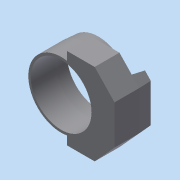
# Autodesk Inventor part: cellSTORM_inverted_objectiveadapter
Saved by Autodesk Inventor 2019.4 (Build 234330000, 330)
## iProperties
Created: 2020-11-10
Part Number: cellSTORM_inverted_objectiveadapter
Material: Generic
Document SubType Name: Modeling
Designer: diederichbenedict
Density: 1 g/cm^3
Appearance: Default
Author: diederichbenedict
Autodesk Inventor part; units mm, degrees
ref_plane "YZ Plane" through (0, 0, 0) normal (1, 0, 0) x (0, 1, 0)
ref_plane "XZ Plane" through (0, 0, 0) normal (0, 1, 0) x (-1, 0, 0)
ref_plane "XY Plane" through (0, 0, 0) normal (0, 0, 1) x (1, 0, 0)
sketch "Sketch1" plane through (0, 0, 0) normal (0, 0, 1) x (1, 0, 0)
  arc A0 (-5.5118, -5.25) -> (-5.5118, 21.75) centre (-8.0118, 8.25) ccw projected
  circle A1 centre (-7.8118, 8.25) radius 10 construction
  circle A2 centre (-7.8118, 8.25) radius 12.15 construction
  line L0 (-5.5118, -8.25) -> (-5.5118, -5.25) construction
  line L1 (7.4882, -8.25) -> (-5.5118, -8.25) construction
  line L2 (11.0118, -4.7265) -> (7.4882, -8.25) construction
  line L3 (11.0118, -4.7265) -> (11.0118, 21.2265) construction
  line L4 (11.0118, 21.2265) -> (7.4882, 24.75) construction
  line L5 (7.4882, 24.75) -> (-5.5118, 24.75) construction
  line L6 (-5.5118, 24.75) -> (-5.5118, 21.75) construction
  arc A3 (-5.5118, -5.25) -> (-5.5118, 21.75) centre (-8.0118, 8.25) ccw construction
  circle A4 centre (-7.8118, 8.25) radius 12.25
  circle A5 centre (-7.8118, 8.25) radius 13.25
  line L7 (-5.5118, 21.2989) -> (-5.5118, 24.75)
  line L8 (-5.5118, 24.75) -> (5.7178, 24.75)
  line L9 (5.7178, 24.75) -> (5.7178, -8.25)
  line L10 (5.7178, 24.75) -> (38.7178, 24.75) construction
  line L11 (5.7178, -8.25) -> (-5.5118, -8.25)
  line L12 (-5.5118, -8.25) -> (-5.5118, -4.7989)
  line L13 (13.7178, 16.3622) -> (5.7178, 16.3622)
  line L14 (5.7178, 16.3622) -> (5.7178, 0.5675)
  line L15 (5.7178, 0.5675) -> (13.7178, 0.5675)
  line L16 (13.7178, 0.5675) -> (13.7178, 16.3622)
  line L17 (13.7178, 16.3622) -> (5.7178, 0.5675) construction
  line L18 (5.7178, 16.3622) -> (13.7178, 0.5675) construction
  line L19 (13.7178, 0.5675) -> (5.7178, -8.25)
  line L20 (13.7178, 16.3622) -> (5.7178, 24.75)
  point P0 (0, 0)
  point P1 (9.7178, 8.4649)
  dimension "d0" = 24.5
  dimension "d1" = 26.5
  dimension "d2" = 90
  dimension "d7" = 8
  constraints: 28 end point, 3 horizontal, 3 perpendicular, 3 point on line, 2 centre point, 2 coincident, 2 midpoint, 2 parallel, 2 point on circle, 1 collinear
  measures "d0" diameter of A4
  measures "d1" diameter of A5
  measures "d2" angle of L9 L10
  measures "d7" distance between parallel lines of L16 L14
extrude "Extrusion1" add sketch "Sketch1" along normal blind 10
sketch "Sketch2" plane through (0, 0, 0) normal (0, 0, -1) x (-1, 0, 0)
  line L0 (-5.7178, -8.25) -> (-5.7178, 24.75) projected
  circle A0 centre (7.8118, 8.25) radius 12.25 projected
  line L1 (5.5118, -8.25) -> (-5.7178, -8.25) projected
  line L2 (5.5118, -4.7989) -> (5.5118, -8.25) projected
  arc A1 (5.5118, -4.7989) -> (5.5118, 21.2989) centre (7.8118, 8.25) ccw projected
  line L3 (5.5118, 24.75) -> (5.5118, 21.2989) projected
  line L4 (-5.7178, 24.75) -> (5.5118, 24.75) projected
  circle A2 centre (7.8118, 8.25) radius 13.25
  line L5 (-13.7178, 16.3622) -> (-5.7178, 24.75) projected
  line L6 (-13.7178, 0.5675) -> (-13.7178, 16.3622) projected
  line L7 (-5.7178, -8.25) -> (-13.7178, 0.5675) projected
  line L8 (-13.7178, 16.3622) -> (-5.7178, 24.75) projected
  line L9 (-13.7178, 0.5675) -> (-13.7178, 16.3622) projected
  line L10 (-5.7178, -8.25) -> (-13.7178, 0.5675) projected
  line L11 (-11.0118, 21.2265) -> (-11.0118, -4.7265) construction
  line L12 (-10.6722, 19.5554) -> (-10.6722, -2.7892)
  line L13 (-5.7178, -8.25) -> (-13.7178, 0.5675) projected
  line L14 (-10.6722, 19.5554) -> (11.6724, 19.5554) construction
  point P0 (0, 0)
  dimension "d8" = 90
  constraints: 4 end point, 2 point on line, 1 centre point, 1 coincident, 1 horizontal, 1 perpendicular
  measures "d8" angle of L12 L14
extrude "Extrusion2" add sketch "Sketch2" along normal blind 3 draft -5 contours L7 L6 L5 L12 | A2 A1
body "Solid1"
